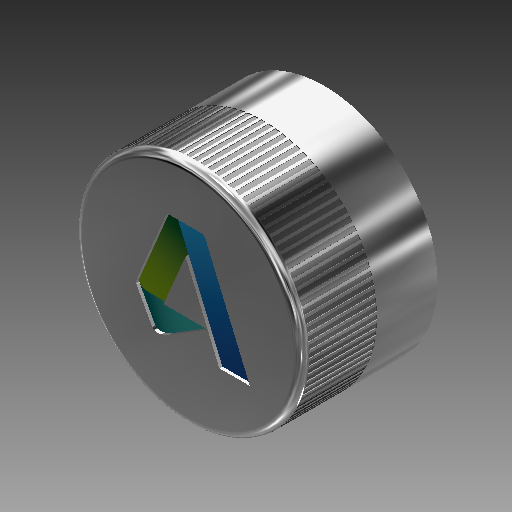
# Autodesk Inventor part: 308-17
Saved by Autodesk Inventor 2019 (Build 230136000, 136)
## iProperties
Company: Autodesk Inc.
Created: 2012-01-24
Part Number: 308-17
Material: Steel
Document SubType Name: Modeling
Designer: Autodesk Inc.
Mass: 4.82131 g
Surface Area: 11.3465 cm^2
Volume: 0.614179 cm^3
Density: 7.85 g/cm^3
Appearance: Chrome - Polished
Author: Inventor
Autodesk Inventor part; units mm, degrees
note: some values were not read from the file. Chosen so that the rebuilt part matches the saved one: direction of "Emboss1"; direction of "Emboss2".
ref_plane "YZ Plane" through (0, 0, 0) normal (1, 0, 0) x (0, 1, 0)
sketch "Sketch1" plane through (0, 0, 0) normal (0, 0, 1) x (1, 0, 0)
  circle A0 centre (0, 0) radius 7.5
  dimension "d0" = 15
  constraints: 1 centre point, 1 coincident
  measures "d0" diameter of A0
extrude "Extrusion1" add sketch "Sketch1" along normal blind 9
sketch "Sketch2" plane through (0, 0, 0) normal (0, 0, -1) x (-1, 0, 0)
  circle A0 centre (0, -0.2224) radius 7
  dimension "d3" = 14
  constraints: 1 centre point
  measures "d3" diameter of A0
extrude "Extrusion2" cut sketch "Sketch2" against normal blind 1.6
hole "Hole1" at (0, -0.2224, 1.6) direction (0, 0, 1) diameter 11.835 depth 6.5 thread size "M14x2" class "6H" standard "ISO Metric profile"
ref_plane "Work Plane1" through (0, 0, 4) normal (0, 0, 1) x (1, 0, 0)
split_face "Split1"
fillet "Fillet1" radius 0.5 1 edges at (-7.5, 0, 9)
ref_plane "Work Plane2" through (0, -7.5, 0) normal (0, 1, 0) x (-1, 0, 0)
sketch "Sketch3" plane through (0, -7.5, 0) normal (0, 1, 0) x (-1, 0, 0)
  line L0 (-7.5, 4) -> (7.5, 4) projected
  line L1 (7.5, 8.5) -> (-7.5, 8.5) projected
  line L2 (-0.15, 4) -> (0.15, 4)
  line L3 (0.15, 4) -> (0.15, 8.5)
  line L4 (0.15, 8.5) -> (-0.15, 8.5)
  line L5 (-0.15, 8.5) -> (-0.15, 4)
  point P0 (0, 0)
  dimension "d31" = 0.3
  dimension "d32" = 4.5
  dimension "d33" = 0.15
  dimension "d34" = 4
  constraints: 8 end point, 2 parallel, 1 horizontal, 1 perpendicular
  measures "d31" distance of L3.end L4.end
  measures "d32" distance of L2.end L3.end
  measures "d33" horizontal distance of L2.start point (0, 0)
  measures "d34" distance from line of point (0, 0) L2
emboss "Emboss1" sketch "Sketch3" operation cut depth 0.05 direction (0, 1, 0)
pattern_circular "Circular Pattern1" count 100 over 360 about axis through (0, 0, 0) along (0, 0, 1) of "Emboss1"
sketch "Sketch5" plane through (0, 0, 9) normal (0, 0, 1) x (1, 0, 0)
  line L0 (-8.0791, 6.8575) -> (8.8043, 6.8575) construction
  line L1 (8.8043, 6.8575) -> (8.8043, -5.805) construction
  line L2 (8.8043, -5.805) -> (-8.0791, -5.805) construction
  line L3 (-8.0791, -5.805) -> (-8.0791, 6.8575) construction
  line L4 (1.2928, -1.31) -> (-1.2437, -2.8905)
  line L5 (-3.3877, -1.096) -> (-2.3801, -2.9531)
  line L6 (-1.4496, 3.8561) -> (-3.3774, -0.7279)
  line L7 (-1.2125, 3.9999) -> (0.8907, 3.9999)
  line L8 (4.0941, -3.1373) -> (1.1488, 3.8288)
  line L9 (4.0941, -3.1373) -> (2.0768, -3.1373)
  line L10 (2.0768, -3.1373) -> (-0.1567, 2.1401)
  line L11 (-0.1567, 2.1401) -> (-1.616, -1.31)
  line L12 (-1.616, -1.31) -> (1.2928, -1.31)
  arc A0 (-2.3801, -2.9531) -> (-2.0852, -3.1375) centre (-2.0591, -2.7677) ccw
  arc A1 (-2.0852, -3.1375) -> (-1.6482, -3.0666) centre (-2.0172, -2.1745) ccw
  line L13 (-1.6482, -3.0666) -> (-1.2437, -2.8905)
  arc A2 (1.1488, 3.8288) -> (0.8907, 3.9999) centre (0.8907, 3.7197) ccw
  arc A3 (-1.2125, 3.9999) -> (-1.4496, 3.8561) centre (-1.1868, 3.6903) ccw
  arc A4 (-3.3774, -0.7279) -> (-3.3877, -1.096) centre (-2.908, -0.9253) ccw
  point P0 (0, 0)
  constraints: 20 end point, 10 point on circle, 5 centre point, 4 tangent, 2 horizontal, 1 parallel, 2 other
emboss "Emboss2" sketch "Sketch5" operation cut depth 0.2 direction (0, 0, -1)
decal "Decal1"
equation "\"d33\" = 0.5 * d31"
body "Solid1"
